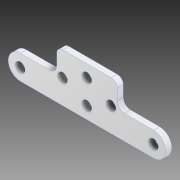
# Autodesk Inventor part: Front - Back Bearing Plate (R4)
Saved by Autodesk Inventor 2022 (Build 260153000, 153)
## iProperties
Created: 2020-09-04
Part Number: Front - Back Bearing Plate (R4)
Material: Aluminum 6061
Document SubType Name: Modeling
Density: 2.7 g/cm^3
Appearance: Aluminum - Flat
Mass: 11.146 g
Surface Area: 35.3191 cm^2
Volume: 4.12814 cm^3
Autodesk Inventor part; units mm, degrees
ref_plane "YZ Plane" through (0, 0, 0) normal (1, 0, 0) x (0, 1, 0)
ref_plane "XZ Plane" through (0, 0, 0) normal (0, 1, 0) x (-1, 0, 0)
ref_plane "XY Plane" through (0, 0, 0) normal (0, 0, 1) x (1, 0, 0)
sketch "Sketch1" plane through (0, 0, 0) normal (0, 0, 1) x (1, 0, 0)
  line L0 (25.4, 6.35) -> (-25.4, 6.35)
  line L1 (-25.4, 6.35) -> (-25.4, -6.35)
  line L2 (-25.4, -6.35) -> (25.4, -6.35)
  line L3 (25.4, -6.35) -> (25.4, 6.35)
  line L4 (25.4, 6.35) -> (-25.4, -6.35) construction
  line L5 (-25.4, 6.35) -> (25.4, -6.35) construction
  line L6 (-25.4, 6.35) -> (-34.925, 6.35)
  line L7 (-34.925, -6.35) -> (-25.4, -6.35)
  arc A0 (-34.925, 6.35) -> (-34.925, -6.35) centre (-34.925, 0) ccw
  circle A1 centre (-34.925, 0) radius 2.4892
  circle A2 centre (-34.925, 0) radius 9.525 construction
  line L8 (0, 0) -> (0, 12.7) construction
  line L9 (25.4, 6.35) -> (34.925, 6.35)
  line L10 (34.925, -6.35) -> (25.4, -6.35)
  arc A3 (34.925, -6.35) -> (34.925, 6.35) centre (34.925, 0) ccw
  circle A4 centre (34.925, 0) radius 2.4892
  line L11 (-15.875, 19.05) -> (15.875, 19.05)
  line L12 (15.875, 19.05) -> (15.875, 6.35)
  line L13 (15.875, 6.35) -> (-15.875, 6.35)
  line L14 (-15.875, 6.35) -> (-15.875, 19.05)
  line L15 (-15.875, 19.05) -> (15.875, 6.35) construction
  line L16 (15.875, 19.05) -> (-15.875, 6.35) construction
  circle A5 centre (0, 0) radius 2.4892
  circle A6 centre (0, 12.7) radius 2.4892
  circle A7 centre (-12.7, 6.35) radius 2.4892
  circle A8 centre (12.7, 6.35) radius 2.4892
  line L17 (-12.7, 6.35) -> (12.7, 6.35)
  point P0 (-15.875, 6.35)
  point P1 (0, 12.7)
  point P2 (0, 6.35)
  dimension "d1" = 50.8
  dimension "d3" = 4.9784
  dimension "d4" = 19.05
  dimension "d5" = 12.7
  dimension "d18" = 4.9784
  dimension "d21" = 12.7
  dimension "d22" = 25.4
  dimension "d26" = 31.75
  constraints: 36 end point, 9 centre point, 6 midpoint, 5 coincident, 4 horizontal, 4 parallel, 4 point on circle, 4 symmetric about line, 3 equal radius, 3 point on line, 3 tangent, 2 perpendicular, 1 collinear, 1 vertical, 1 vertical alignment, 2 other
  measures "d1" distance between parallel lines of L3 L1
  measures "d3" diameter of A1
  measures "d4" diameter of A2
  measures "d5" diameter of A0
  measures "d18" diameter of A5
  measures "d21" distance of L8.start L8.end
  measures "d22" distance of L17.start L17.end
  measures "d26" distance between parallel lines of L12 L14
extrude "Extrusion1" add sketch "Sketch1" along normal blind 3.175 contours L3 L2 L1 L0 A7 A8 | L9 A3 L10 L3 | L0 A8 A7 L14 L11 L12 | L7 A0 L6 L1
fillet "Fillet1" radius 3.81 2 edges at (15.875, 6.35, 1.5875) (-15.875, 6.35, 1.5875)
fillet "Fillet1" radius 3.175 2 edges at (15.875, 19.05, 1.5875) (-15.875, 19.05, 1.5875)
body "Solid1"
